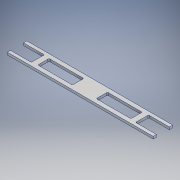
# Autodesk Inventor part: top
Saved by Autodesk Inventor 2017 (Build 210142000, 142)
## iProperties
Created: 2016-09-24
Part Number: top
Material: Aluminum 6061
Document SubType Name: Modeling
Designer: Kevin G
Density: 2.7 g/cm^3
Appearance: Aluminum - Flat
Author: Kevin G
Autodesk Inventor part; units mm, degrees
ref_plane "YZ Plane" through (0, 0, 0) normal (1, 0, 0) x (0, 1, 0)
ref_plane "XZ Plane" through (0, 0, 0) normal (0, 1, 0) x (-1, 0, 0)
ref_plane "XY Plane" through (0, 0, 0) normal (0, 0, 1) x (1, 0, 0)
sketch "Sketch1" plane through (0, 0, 0) normal (0, 0, 1) x (1, 0, 0)
  arc A0 (-179.9924, 22) -> (-183.6588, 16.912) centre (-179.5223, 17.7962) ccw
  arc A1 (-183.6588, -17.77) -> (-179.4288, -22) centre (-179.4288, -17.77) ccw
  arc A2 (-48.2588, 16.912) -> (-52.4305, 22) centre (-52.4009, 17.7701) ccw
  arc A3 (-52.9925, -22) -> (-48.2588, -17.77) centre (-52.4887, -17.8001) ccw
  line L0 (-52.4305, 22) -> (-179.9924, 22)
  line L1 (-52.9925, -22) -> (-179.4288, -22)
  line L2 (-48.2588, -17.77) -> (-48.2588, 16.912)
  line L3 (-183.6588, -17.77) -> (-183.6588, 16.912)
  line L4 (-286.5288, -25.829) -> (-208.4238, -25.829)
  line L5 (-286.5288, 24.971) -> (-208.4238, 24.971)
  line L6 (-205.2488, 21.796) -> (-205.2488, -22.654)
  arc A4 (-205.2488, 21.796) -> (-208.4238, 24.971) centre (-208.4238, 21.796) ccw
  arc A5 (-208.4238, -25.829) -> (-205.2488, -22.654) centre (-208.4238, -22.654) ccw
  arc A6 (44.1612, -17.77) -> (48.3912, -22) centre (48.3912, -17.77) ccw
  arc A7 (47.8276, 22) -> (44.1612, 16.912) centre (48.2978, 17.7962) ccw
  line L7 (44.1612, -17.77) -> (44.1612, 16.912)
  line L8 (204.3262, 25.4) -> (282.4312, 25.4)
  line L9 (204.3262, -25.4) -> (282.4312, -25.4)
  line L10 (174.8276, -22) -> (48.3912, -22)
  line L11 (175.3896, 22) -> (47.8276, 22)
  arc A8 (179.5612, 16.912) -> (175.3896, 22) centre (175.4192, 17.7701) ccw
  line L12 (179.5612, -17.77) -> (179.5612, 16.912)
  arc A9 (174.8276, -22) -> (179.5612, -17.77) centre (175.3313, -17.8001) ccw
  arc A10 (201.1512, -22.225) -> (204.3262, -25.4) centre (204.3262, -22.225) ccw
  arc A11 (204.3262, 25.4) -> (201.1512, 22.225) centre (204.3262, 22.225) ccw
  line L13 (201.1512, 22.225) -> (201.1512, -22.225)
  line L14 (-286.5288, 38.1) -> (282.4312, 38.1)
  line L15 (-286.5288, -38.1) -> (282.4312, -38.1)
  line L16 (282.4312, 38.1) -> (282.4312, 25.4)
  line L17 (282.4312, -25.4) -> (282.4312, -38.1)
  line L18 (-286.5288, 38.1) -> (-286.5288, 24.971)
  line L19 (-286.5288, -25.829) -> (-286.5288, -38.1)
  dimension "d0" = 135.4
  dimension "d1" = 44
  dimension "d8" = 78.105
  dimension "d13" = 50.8
  dimension "d14" = 44.45
  dimension "d15" = 21.59
  dimension "d18" = 135.4
  dimension "d19" = 44
  dimension "d20" = 78.105
  dimension "d21" = 50.8
  dimension "d26" = 568.96
  dimension "d33" = 21.59
  constraints: 40 end point, 28 point on circle, 12 centre point, 8 vertical, 7 horizontal, 2 perpendicular, 1 parallel, 1 point on line
  measures "d0" distance between parallel lines of L2 L3
  measures "d1" distance between parallel lines of L1 L0
  measures "d8" distance of L4.start L4.end
  measures "d13" distance between parallel lines of L4 L5
  measures "d14" distance of L6.start L6.end
  measures "d15" distance between parallel lines of L3 L6
  measures "d18" distance between parallel lines of L12 L7
  measures "d19" distance between parallel lines of L10 L11
  measures "d20" distance of L9.start L9.end
  measures "d21" distance between parallel lines of L9 L8
  measures "d26" distance of L14.end L14.start
  measures "d33" distance between parallel lines of L13 L12
extrude "Extrusion2" add sketch "Sketch1" along normal blind 9.525
body "Solid2"
